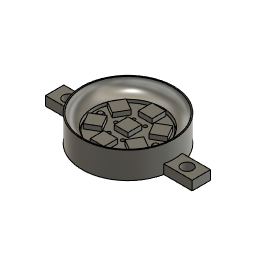
Seven LED Insert (Autodesk Fusion 360 design; units mm, degrees)
part number: arr-00-003
Autodesk Fusion 360 part; units mm, degrees
sketch "Sketch1" plane through (0, 0, 0) normal (0, 1, 0) x (1, 0, 0) in component "Seven LED Mount"
  circle A0 centre (0, 0) radius 11.9062
  circle A1 centre (0, 0) radius 15.875
  circle A2 centre (0, 0) radius 15.4781
  circle A3 centre (0, 0) radius 12.7
  line L0 (25.4, 3.175) -> (15.5543, 3.175)
  line L1 (25.4, 3.175) -> (25.4, -3.175)
  line L2 (25.4, -3.175) -> (15.5543, -3.175)
  line L3 (-15.5543, 3.175) -> (-25.4, 3.175)
  line L4 (-25.4, 3.175) -> (-25.4, -3.175)
  line L5 (-25.4, -3.175) -> (-15.5543, -3.175)
  circle A4 centre (-20.4771, 0) radius 1.9844
  circle A5 centre (20.4771, 0) radius 1.9844
  dimension "d1" = 23.8125
  dimension "d2" = 31.75
  dimension "d3" = 30.9563
  dimension "d4" = 25.4
  dimension "d5" = 3.9688
  dimension "d6" = 3.9688
  constraint coincident A0.centre A1.centre
  constraint concentric A1 A2
  constraint concentric A2 A3
  constraint coincident A1 L0.end
  constraint horizontal L0
  constraint perpendicular L0 L1
  constraint coincident A1 L2.end
  constraint perpendicular L1 L2
  constraint coincident A1 L3.start
  constraint parallel L2 L3
  constraint perpendicular L3 L4
  constraint coincident A1 L5.end
  constraint perpendicular L4 L5
  measures "d1" diameter of A0
  measures "d2" diameter of A1
  measures "d3" diameter of A2
  measures "d4" diameter of A3
  measures "d5" diameter of A4
  measures "d6" diameter of A5
extrude "Extrude1" add sketch "Sketch1" along normal blind 3.175 contours A0 | A1 | A1 L0 L1 L2 | A1 L3 L4 L5 | A2 | A3 makes body 1 in component "Seven LED Mount"
extrude "Extrude2" add sketch "Sketch1" along normal blind 4.7625 contours A3 bodies 1 in component "Seven LED Mount"
extrude "Extrude3" add sketch "Sketch1" along normal blind 4.7625 contours A1 | A2 bodies 1 in component "Seven LED Mount"
extrude "Extrude4" add sketch "Sketch1" along normal blind 9.1281 contours A1 bodies 1 in component "Seven LED Mount"
sketch "Sketch2" plane through (0, 0, 0) normal (0, 0, 1) x (1, 0, 0) in component "Seven LED Mount"
  arc A0 (-15.4781, 9.1281) -> (-11.9062, 4.7625) centre (-11.0426, 9.1132) ccw
  line L0 (-15.4781, 9.1281) -> (-15.4781, 4.7625)
  line L1 (-15.4781, 4.7625) -> (-11.9062, 4.7625)
  point P0 (-15.4781, 9.1281)
  point P1 (-11.9062, 4.7625)
  constraint coincident P1 A0.end
  constraint coincident P0 A0.start
  constraint vertical L0
  constraint perpendicular L0 L1
sweep "Sweep1" add profiles "Sketch2" along 1 edges at (-11.9062, 4.7625, 0) section 1 on bodies 1 bodies 1 in component "Seven LED Mount"
sketch "Sketch3" plane through (0, 3.175, 0) normal (0, 1, 0) x (-1, 0, 0) in component "Seven LED Mount"
  circle A0 centre (0, 0) radius 11.9062
  circle A1 centre (9.6083, 0) radius 0.7649
  circle A2 centre (-9.6319, 0) radius 0.762
  point P0 (11.9062, 0)
  point P1 (-11.9062, 0)
  dimension "d22" = 1.5297
  dimension "d24" = 1.524
  measures "d22" diameter of A1
  measures "d24" diameter of A2
extrude "Extrude5" add sketch "Sketch3" along normal blind 0.7937 contours A1 | A2 bodies 1 in component "Seven LED Mount"
sketch "Sketch4" plane through (0, 3.175, 0) normal (0, 1, 0) x (-1, 0, 0) in component "Seven LED Mount"
  circle A0 centre (-9.6319, 0) radius 0.762
  circle A1 centre (9.6083, 0) radius 0.7649
  circle A2 centre (0, 0) radius 11.9062
  circle A3 centre (0, 0) radius 8.7313
  dimension "d27" = 17.4625
  constraint coincident A2.centre A3.centre
  measures "d27" diameter of A3
extrude "Extrude6" cut sketch "Sketch4" against normal blind 3.175 contours A3 bodies 1 in component "Seven LED Mount"
extrude "Extrude7" add 2 faces at (-9.3786, 3.9688, 0.2271) (9.6269, 3.9688, -0.1921) along direction (0, 1, 0) blind 0.3969 on bodies 1 bodies 1 in component "Seven LED Mount"
sketch "Sketch1 (2)" plane through (0, 0, 0) normal (0, 1, 0) x (1, 0, 0) in component "Seven LED Board"
  circle A0 centre (76.2, 0) radius 11.5094
  circle A1 centre (66.6619, 0) radius 1.143
  circle A2 centre (85.8449, 0) radius 1.143
  line L0 (73.8187, 10.7156) -> (78.5812, 10.7156)
  line L1 (78.5812, 10.7156) -> (78.5812, 5.9531)
  line L2 (78.5812, 5.9531) -> (73.8187, 5.9531)
  line L3 (73.8187, 5.9531) -> (73.8187, 10.7156)
  line L4 (69.8538, 0.9143) -> (65.7294, 3.2956)
  line L5 (72.2351, 5.0388) -> (69.8538, 0.9143)
  line L6 (68.1106, 7.42) -> (72.2351, 5.0388)
  line L7 (65.7294, 3.2956) -> (68.1106, 7.42)
  line L8 (72.2351, -5.0388) -> (68.1106, -7.42)
  line L9 (69.8538, -0.9143) -> (72.2351, -5.0388)
  line L10 (65.7294, -3.2956) -> (69.8538, -0.9143)
  line L11 (68.1106, -7.42) -> (65.7294, -3.2956)
  line L12 (78.5812, -5.9531) -> (78.5812, -10.7156)
  line L13 (73.8187, -5.9531) -> (78.5812, -5.9531)
  line L14 (73.8187, -10.7156) -> (73.8187, -5.9531)
  line L15 (78.5812, -10.7156) -> (73.8187, -10.7156)
  line L16 (82.5462, -0.9143) -> (86.6706, -3.2956)
  line L17 (80.1649, -5.0388) -> (82.5462, -0.9143)
  line L18 (84.2894, -7.42) -> (80.1649, -5.0388)
  line L19 (86.6706, -3.2956) -> (84.2894, -7.42)
  line L20 (80.1649, 5.0388) -> (84.2894, 7.42)
  line L21 (82.5462, 0.9143) -> (80.1649, 5.0388)
  line L22 (86.6706, 3.2956) -> (82.5462, 0.9143)
  line L23 (84.2894, 7.42) -> (86.6706, 3.2956)
  line L24 (78.5812, 2.3813) -> (78.5812, -2.3813)
  line L25 (78.5812, -2.3813) -> (73.8187, -2.3813)
  line L26 (73.8187, -2.3813) -> (73.8187, 2.3813)
  line L27 (73.8187, 2.3813) -> (78.5812, 2.3813)
  circle A3 centre (73.9981, 4.1267) radius 0.5953
  circle A4 centre (78.0651, 4.0807) radius 0.5953
  circle A5 centre (73.7223, -4.1453) radius 0.5953
  circle A6 centre (78.3408, -4.0074) radius 0.5953
  circle A7 centre (71.8382, 0.1975) radius 0.5953
  point P0 (76.2, 10.7156)
  dimension "d32" = 23.0187
  dimension "d35" = 2.286
  dimension "d36" = 2.286
  dimension "d37" = 4.7625
  dimension "d38" = 4.7625
  dimension "d41" = 360
  dimension "d44" = 4.7625
  dimension "d45" = 4.7625
  dimension "d50" = 1.1906
  dimension "d51" = 1.1906
  dimension "d52" = 1.1906
  dimension "d53" = 1.1906
  dimension "d54" = 1.1906
  constraint horizontal L0
  constraint vertical L1
  constraint horizontal L2
  constraint vertical L3
  constraint midpoint L0 P0
  constraint vertical L24
  constraint perpendicular L24 L25
  constraint perpendicular L25 L26
  constraint perpendicular L24 L27
  measures "d32" diameter of A0
  measures "d35" diameter of A1
  measures "d36" diameter of A2
  measures "d37" distance of L0.start L0.end
  measures "d38" distance of L0.start L2.end
  measures "d44" distance of L24.start L24.end
  measures "d45" distance of L24.end L25.end
  measures "d50" diameter of A3
  measures "d51" diameter of A4
  measures "d52" diameter of A5
  measures "d53" diameter of A6
  measures "d54" diameter of A7
extrude "Extrude1'" add sketch "Sketch1 (2)" along normal blind 0.7937 separate body makes body 2 in component "Seven LED Board"
extrude "Extrude2'" add sketch "Sketch1 (2)" along normal blind 2.3813 contours L0 L1 L2 L3 | L4 L5 L6 L7 | L8 L9 L10 L11 | L12 L13 L14 L15 | L16 L17 L18 L19 | L20 L21 L22 L23 | L24 L25 L26 L27 bodies 2 in component "Seven LED Board"
component "Seven LED Mount" placed x (1, 0, 0) y (0, 1, 0) z (0, 0, 1) at (0, 0, 0)
component "Seven LED Board" placed x (1, 0, 0) y (0, 1, 0) z (0, 0, 1) at (-76.2, 3.175, 0)
equation "d1 = ( 15 / 16 ) * 1 in"
equation "d3 = 1 7/32\""
equation "d5 = ( 5 / 32 ) * 1 in"
equation "d6 = ( 5 / 32 ) * 1 in"
equation "d7 = ( 1 / 8 ) * 1 in"
equation "d9 = ( 3 / 16 ) * 1 in"
equation "d11 = ( 3 / 16 ) * 1 in"
equation "d13 = ( 23 / 64 ) * 1 in"
equation "d25 = ( 1 / 32 ) * 1 in"
equation "d27 = ( 11 / 16 ) * 1 in"
equation "d28 = ( -1 / 8 ) * 1 in"
equation "d30 = ( 1 / 64 ) * 1 in"
equation "d32 = ( 29 / 32 ) * 1 in"
equation "d37 = ( 3 / 16 ) * 1 in"
equation "d38 = ( 3 / 16 ) * 1 in"
equation "d44 = ( 3 / 16 ) * 1 in"
equation "d45 = ( 3 / 16 ) * 1 in"
equation "d46 = ( 1 / 32 ) * 1 in"
equation "d48 = ( 3 / 32 ) * 1 in"
equation "d50 = ( 3 / 64 ) * 1 in"
equation "d51 = ( 3 / 64 ) * 1 in"
equation "d52 = ( 3 / 64 ) * 1 in"
equation "d53 = ( 3 / 64 ) * 1 in"
equation "d54 = ( 3 / 64 ) * 1 in"
